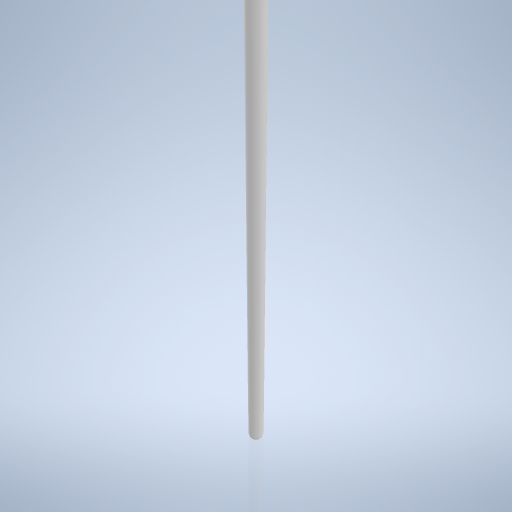
# Autodesk Inventor part: ventri-einsatz
Saved by Autodesk Inventor 2024.2 (Build 282272000, 272)
## iProperties
Created: 2024-04-30
Part Number: ventri-einsatz
Material: Generisch
Document SubType Name: Modeling
Designer: Fabri
Density: 1 g/cm^3
Appearance: Vorgabe
Author: Fabri
Autodesk Inventor part; units mm, degrees
ref_plane "YZ Plane" through (0, 0, 0) normal (1, 0, 0) x (0, 1, 0)
ref_plane "XZ Plane" through (0, 0, 0) normal (0, 1, 0) x (-1, 0, 0)
ref_plane "XY Plane" through (0, 0, 0) normal (0, 0, 1) x (1, 0, 0)
sketch "Skizze2" plane through (0, 0, 0) normal (0, 1, 0) x (-1, 0, 0)
  arc A0 (1, -1) -> (0, 0) centre (0, -1) ccw
  line L0 (1, -1) -> (1, -57)
  arc A1 (0, -58) -> (1, -57) centre (0, -57) ccw
  line L1 (0, -58) -> (0, 0)
  dimension "d3" = 1
  dimension "d4" = 58
  dimension "d5" = 2
  constraints: 4 end point, 4 point on circle, 2 centre point, 2 vertical, 1 equal radius, 1 tangent, 1 vertical alignment
  measures "d3" radius of A0
  measures "d4" distance of L1.start L1.end
  measures "d5" diameter of L0 L1
revolve "Umdrehung1" add sketch "Skizze2" angle 360 about axis through (0, 0, -58) along (0, 0, 1)
